potar_v1 (Autodesk Fusion 360 design; units mm, degrees)
Autodesk Fusion 360 part; units mm, degrees
sketch "Esquisse1" plane through (0, 0, 0) normal (0, 0, 1) x (1, 0, 0)
  line L0 (-8.5, 0) -> (8.5, 0)
  line L1 (8.5, 0) -> (8.5, -11)
  line L2 (8.5, -11) -> (-8.5, -11) construction
  line L3 (-8.5, -11) -> (-8.5, 0)
  circle A0 centre (0, 0) radius 3.5
  arc A1 (8.5, 0) -> (-8.5, 0) centre (0, 0) ccw
  line L4 (10.5, 0) -> (10.5, -13)
  line L5 (10.5, -13) -> (-10.5, -13)
  line L6 (-10.5, -13) -> (-10.5, 0)
  arc A2 (10.5, 0) -> (-10.5, 0) centre (0, 0) ccw
  line L7 (-8.5, -11) -> (-8.5, -13)
  line L8 (8.5, -11) -> (8.5, -13)
  line L9 (10.5, -13) -> (16.5, -13)
  line L10 (16.5, -13) -> (16.5, 0)
  line L11 (16.5, 0) -> (10.5, 0)
  line L12 (10.5, 0) -> (10.5, -13)
  line L13 (0, 0) -> (0, -13) construction
  line L14 (-16.5, -13) -> (-16.5, 0)
  line L15 (-10.5, -13) -> (-16.5, -13)
  line L16 (-16.5, 0) -> (-10.5, 0)
  circle A3 centre (13.5, -6.5) radius 1.7
  line L17 (16.5, -6.5) -> (10.5, -6.5) construction
  line L18 (13.5, 0) -> (13.5, -13) construction
  circle A4 centre (-13.5, -6.5) radius 1.7
  dimension "d1" = 17
  dimension "d2" = 17
  dimension "d3" = 11
  dimension "d4" = 7
  dimension "d5" = -2
  dimension "d6" = 6
  dimension "d7" = 3.4
  constraint coincident A0.centre A1.centre
  constraint horizontal L0
  constraint vertical L1
  constraint horizontal L2
  constraint vertical L3
  constraint coincident A0.centre L0
  constraint coincident L5 L7.end
  constraint perpendicular L5 L7
  constraint coincident L5 L8.end
  constraint perpendicular L5 L8
  constraint horizontal L9
  constraint vertical L10
  constraint horizontal L11
  constraint vertical L12
  constraint collinear L0 L11
  constraint midpoint L5 L13.end
  constraint symmetric L4.end L13 L5.end
  constraint symmetric L9.end L13 L14.start
  constraint symmetric L10.end L13 L14.end
  constraint symmetric L4.start L13 L6.end
  constraint midpoint L10 L17.start
  constraint midpoint L12 L17.end
  constraint midpoint L11 L18.start
  constraint midpoint L9 L18.end
  constraint coincident A3.centre L18
  constraint coincident A3.centre L17
  constraint symmetric L13 A3 A4
  measures "d1" diameter of A1
  measures "d2" distance of L0.start L0.end
  measures "d3" distance of L0.start L2.end
  measures "d4" diameter of A0
  measures "d6" distance of L4.end L9.end
  measures "d7" diameter of A3
extrude "Extrusion1" add sketch "Esquisse1" along normal blind 2 contours L4 L9 L10 L11 L12 | L6 L14 L15 L16 makes body 1 at (-13.4577, -11.3984, 0) makes body 2 at (13.5423, -11.3984, 0)
extrude "Extrusion2" add sketch "Esquisse1" along normal blind 9 contours L1 L3 A1 L4 L5 L6 A2 L7 L8 L12 bodies 1 2
sketch "Esquisse2" plane through (0, 0, 9) normal (0, 0, 1) x (-1, 0, 0)
  line L0 (8.5, 13) -> (8.5, 0)
  arc A0 (-8.5, 0) -> (8.5, 0) centre (0, 0) ccw
  line L1 (-8.5, 0) -> (-8.5, 13)
  line L2 (-8.5, 13) -> (-10.5, 13)
  line L3 (-10.5, 13) -> (-10.5, 0)
  arc A1 (-10.5, 0) -> (10.5, 0) centre (0, 0) ccw
  line L4 (10.5, 0) -> (10.5, 13)
  line L5 (10.5, 13) -> (8.5, 13)
  circle A2 centre (0, 0) radius 3.5
  line L6 (-10.5, 13) -> (10.5, 13)
  line L7 (10.5, 13) -> (10.5, 0)
  arc A3 (-10.5, 0) -> (10.5, 0) centre (0, 0) ccw
  line L8 (-10.5, 0) -> (-10.5, 13)
extrude "Extrusion3" add sketch "Esquisse2" along normal blind 2 bodies 1
fillet "Congé1" radius 1 2 edges at (10.5, -6.5, 2) (-10.5, -6.5, 2) on bodies 1
